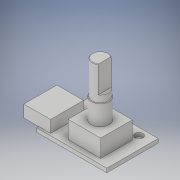
# Autodesk Inventor part: encoder
Saved by Autodesk Inventor 2019 (Build 230136000, 136)
## iProperties
Created: 2019-09-12
Part Number: encoder
Material: Generic
Document SubType Name: Modeling
Designer: assman
Density: 1 g/cm^3
Appearance: Default
Author: assman
Autodesk Inventor part; units mm, degrees
ref_plane "YZ Plane" through (0, 0, 0) normal (1, 0, 0) x (0, 1, 0)
ref_plane "XZ Plane" through (0, 0, 0) normal (0, 1, 0) x (-1, 0, 0)
ref_plane "XY Plane" through (0, 0, 0) normal (0, 0, 1) x (1, 0, 0)
sketch "Sketch1" plane through (0, 0, 0) normal (0, 1, 0) x (-1, 0, 0)
  line L0 (13.125, 9.625) -> (-13.125, 9.625)
  line L1 (-13.125, 9.625) -> (-13.125, -9.625)
  line L2 (-13.125, -9.625) -> (13.125, -9.625)
  line L3 (13.125, -9.625) -> (13.125, 9.625)
  line L4 (13.125, 9.625) -> (-13.125, -9.625) construction
  line L5 (-13.125, 9.625) -> (13.125, -9.625) construction
  circle A0 centre (8.625, -6.925) radius 1.5
  circle A1 centre (-8.625, -6.925) radius 1.5
  line L6 (3.375, 7.625) -> (-8.825, 7.625)
  line L7 (-8.825, 7.625) -> (-8.825, -4.225)
  line L8 (-8.825, -4.225) -> (3.375, -4.225)
  line L9 (3.375, -4.225) -> (3.375, 7.625)
  line L10 (3.375, 7.625) -> (-8.825, -4.225) construction
  line L11 (-8.825, 7.625) -> (3.375, -4.225) construction
  point P0 (0, 0)
  point P1 (-2.725, 1.7)
  dimension "d0" = 26.25
  dimension "d1" = 19.25
  dimension "d2" = 3
  dimension "d3" = 3
  dimension "d5" = 2.7
  dimension "d8" = 4.5
  dimension "d9" = 4.5
  dimension "d11" = 2.7
  dimension "d12" = 12.2
  dimension "d13" = 11.85
  dimension "d14" = 2
  dimension "d15" = 4.3
  constraints: 24 end point, 4 midpoint, 4 parallel, 2 centre point, 2 horizontal, 2 perpendicular
  measures "d0" distance of L2.end L1.end
  measures "d1" distance of L1.end L0.end
  measures "d2" diameter of A0
  measures "d3" diameter of A1
  measures "d5" distance from line of L2 A1.centre
  measures "d8" distance from line of L1 A1.centre
  measures "d9" distance from line of L3 A0.centre
  measures "d11" distance from line of L2 A0.centre
  measures "d12" distance of L8.end L7.end
  measures "d13" distance of L7.end L6.end
  measures "d14" distance between parallel lines of L0 L6
  measures "d15" distance between parallel lines of L1 L7
extrude "Extrusion1" add sketch "Sketch1" against normal blind 1.5
sketch "Sketch2" plane through (0, -1.5, 0) normal (0, -1, 0) x (1, 0, 0)
  line L0 (8.825, -4.225) -> (8.825, 7.625) projected
  line L1 (8.825, 7.625) -> (-3.375, 7.625) projected
  line L2 (-3.375, 7.625) -> (-3.375, -4.225) projected
  line L3 (-3.375, -4.225) -> (8.825, -4.225) projected
  circle A0 centre (8.625, -6.925) radius 1.5 projected
  circle A1 centre (-8.625, -6.925) radius 1.5 projected
  line L4 (-13.125, 9.625) -> (13.125, 9.625) projected
  line L5 (13.125, 9.625) -> (13.125, -9.625) projected
  line L6 (13.125, -9.625) -> (-13.125, -9.625) projected
  line L7 (-13.125, -9.625) -> (-13.125, 9.625) projected
  point P0 (0, 0)
extrude "Extrusion2" add sketch "Sketch2" against normal blind 8.12 contours L3 L2 L1 L0
sketch "Sketch3" plane through (0, 0, 0) normal (0, 1, 0) x (1, 0, 0)
  line L0 (-18.725, -8.875) -> (-8.725, -8.875)
  line L1 (-8.725, -8.875) -> (-8.725, 3.525)
  line L2 (-8.725, 3.525) -> (-18.725, 3.525)
  line L3 (-18.725, 3.525) -> (-18.725, -8.875)
  line L4 (-18.725, -8.875) -> (-8.725, 3.525) construction
  line L5 (-8.725, -8.875) -> (-18.725, 3.525) construction
  line L6 (-13.125, 9.625) -> (-13.125, -9.625) projected
  line L7 (13.125, 9.625) -> (-13.125, 9.625) projected
  point P0 (0, 0)
  point P1 (-13.725, -2.675)
  dimension "d20" = 10
  dimension "d21" = 12.4
  dimension "d22" = 4.4
  dimension "d23" = 18.5
  constraints: 12 end point, 2 midpoint, 2 parallel, 1 horizontal, 1 perpendicular
  measures "d20" distance of L2.end L1.end
  measures "d21" distance of L1.end L0.end
  measures "d22" distance between parallel lines of L6 L1
  measures "d23" distance between parallel lines of L7 L0
extrude "Extrusion3" add sketch "Sketch3" along normal blind 4.5
sketch "Sketch4" plane through (0, 6.62, 0) normal (0, 1, 0) x (1, 0, 0)
  line L0 (8.825, -7.625) -> (8.825, 4.225) projected
  line L1 (8.825, 4.225) -> (-3.375, 4.225) projected
  line L2 (-3.375, 4.225) -> (-3.375, -7.625) projected
  line L3 (-3.375, -7.625) -> (8.825, -7.625) projected
  circle A0 centre (2.725, -1.7) radius 3.35
  point P0 (0, 0)
  dimension "d26" = 6.7
  constraints: 1 centre point
  measures "d26" diameter of A0
extrude "Extrusion4" add sketch "Sketch4" along normal blind 7.5 contours A0
sketch "Sketch5" plane through (2.725, 14.12, 1.7) normal (0, 1, 0) x (1, 0, 0)
  circle A0 centre (0, 0) radius 3.35 projected
  circle A1 centre (0, 0) radius 3
  point P0 (-2.725, 1.7)
  dimension "d29" = 6
  constraints: 1 centre point, 1 coincident
  measures "d29" diameter of A1
extrude "Extrusion5" add sketch "Sketch5" along normal blind 12.56 contours A1
sketch "Sketch6" plane through (2.725, 26.68, 1.7) normal (0, 1, 0) x (1, 0, 0)
  circle A0 centre (0, 0) radius 3 projected
  line L0 (1.7, 2.4718) -> (1.7, -2.4718)
  point P0 (-2.725, 1.7)
  dimension "d32" = 1.7
  constraints: 2 end point, 2 point on circle, 1 vertical
  measures "d32" distance from line of A0.centre L0
extrude "Extrusion6" cut sketch "Sketch6" against normal blind 10 contours A0 L0 picked at (2.1333, 0)
fillet "Fillet1" radius 0.2 1 edges at (-0.275, 26.68, 1.7)
equation "\"d11\" = d5"
body "Solid1"
